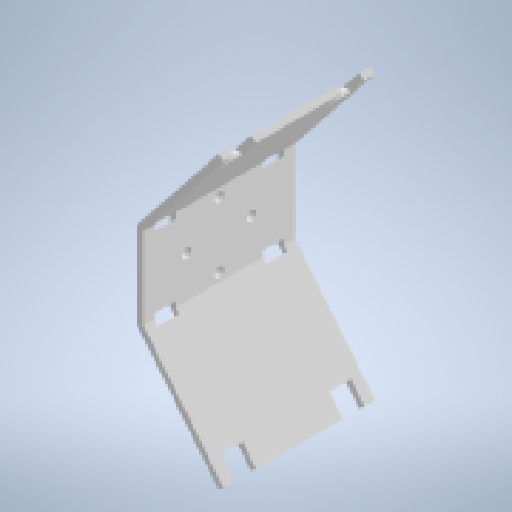
# Autodesk Inventor part: onTubeFixation
Saved by Autodesk Inventor 2024 (Build 280153000, 153)
## iProperties
Created: 2023-07-05
Part Number: onTubeFixation
Material: Generic
Document SubType Name: Sheet Metal
Designer: pablo
Density: 1 g/cm^3
Sheet Metal Rule: Default_mm
Appearance: Default
Author: pablo
Autodesk Inventor part; units mm, degrees
sketch "Sketch2" plane through (0, 0, 0) normal (0, 0, 1) x (1, 0, 0)
  line L0 (0, 0) -> (-40, 50)
  line L1 (-40, 50) -> (-40, 90)
  line L2 (-40, 90) -> (0, 140)
  line L3 (0, 140) -> (0, 0)
  line L4 (-2.3426, 137.0717) -> (0, 135.1977)
  line L5 (-2.3426, 2.9283) -> (0, 4.8023)
  dimension "d4" = 40
  dimension "d5" = 50
  dimension "d6" = 50
  dimension "d7" = 40
  dimension "d11" = 3
  dimension "d12" = 3
  constraints: 12 end point, 4 point on line, 2 perpendicular, 1 parallel, 1 vertical
  measures "d4" distance between parallel lines of L3 L1
  measures "d5" vertical distance of L2.end L1.end
  measures "d6" vertical distance of L0.start L0.end
  measures "d7" distance of L1.end L0.end
  measures "d11" distance of L4.start L4.end
  measures "d12" distance of L5.start L5.end
extrude "Extrusion2" add sketch "Sketch2" along normal mid plane 70 contours L0 L1 L2 L4 L3 L5
shell "Shell1" thickness 3 removed faces 5 at (-13.3333, 63.3333, -35) at (0, 91.7326, 11.6667) at (-13.3333, 63.3333, 35) at (-0.7809, 135.8224, -11.6667) at (-0.7809, 4.1776, 11.6667)
sketch "Sketch4" plane through (-2.3426, 2.9283, -35) normal (-0.7808688, -0.624695, 0) x (0, 0, 1)
  line L0 (0, 0) -> (70, 0) projected
  line L1 (5, 0) -> (15, 0)
  line L2 (15, 0) -> (15, 10)
  line L3 (15, 10) -> (5, 10)
  line L4 (5, 10) -> (5, 0)
  line L5 (55, 0) -> (65, 0)
  line L6 (65, 0) -> (65, 10)
  line L7 (65, 10) -> (55, 10)
  line L8 (55, 10) -> (55, 0)
  line L9 (70, 60.2812) -> (70, 0) projected
  line L10 (0, 0) -> (0, 60.2812) projected
  point P0 (35, -3.75)
  point P1 (70, 54.2734)
  point P2 (0, 54.2734)
  dimension "d54" = 10
  dimension "d55" = 10
  dimension "d56" = 5
  dimension "d57" = 5
  dimension "d58" = 10
  dimension "d59" = 10
  constraints: 16 end point, 4 parallel, 2 horizontal, 2 perpendicular, 2 point on line
  measures "d54" distance between parallel lines of L4 L2
  measures "d55" distance between parallel lines of L6 L8
  measures "d56" distance between parallel lines of L9 L6
  measures "d57" distance between parallel lines of L10 L4
  measures "d58" distance between parallel lines of L0 L3
  measures "d59" distance between parallel lines of L0 L7
extrude "Extrusion3" cut sketch "Sketch4" against normal through all
sketch "Sketch5" plane through (-2.3426, 137.0717, -35) normal (-0.7808688, 0.624695, 0) x (0, 0, 1)
  line L0 (0, 0) -> (70, 0) projected
  line L1 (65, 0) -> (55, 0)
  line L2 (55, 0) -> (55, -10)
  line L3 (55, -10) -> (65, -10)
  line L4 (65, -10) -> (65, 0)
  line L5 (5, 0) -> (15, 0)
  line L6 (15, 0) -> (15, -10)
  line L7 (15, -10) -> (5, -10)
  line L8 (5, -10) -> (5, 0)
  line L9 (0, -60.2812) -> (0, 0) projected
  line L10 (70, 0) -> (70, -60.2812) projected
  point P0 (35, -105.5716)
  point P1 (0, -54.2734)
  point P2 (70, -54.2734)
  point P3 (15, 0)
  point P4 (55, 0)
  dimension "d62" = 5
  dimension "d63" = 5
  dimension "d64" = 10
  dimension "d65" = 10
  dimension "d66" = 10
  constraints: 16 end point, 4 parallel, 3 point on line, 2 horizontal, 2 perpendicular
  measures "d62" distance between parallel lines of L9 L8
  measures "d63" distance between parallel lines of L10 L4
  measures "d64" distance between parallel lines of L2 L4
  measures "d65" distance between parallel lines of L8 L6
  measures "d66" distance between parallel lines of L0 L3
extrude "Extrusion4" cut sketch "Sketch5" against normal through all
fillet "Fillet3" radius 3 4 edges at (-8.5896, 129.2631, -25) (-8.5896, 129.2631, 25) (-8.5896, 10.7369, -25) (-8.5896, 10.7369, 25)
ref_plane "Work Plane1" through (-40, 90, -35) normal (0.3310069, 0.9436283, 0) x (0, 0, -1)
ref_plane "Work Plane2" through (-40, 50, -35) normal (0.3310069, -0.9436283, 0) x (0, 0, 1)
sketch "Sketch8" plane through (-40, 90, -35) normal (0.3310069, 0.9436283, 0) x (0, 0, -1)
  line L0 (0, 0) -> (-70, 0) projected
  line L1 (-65, 0) -> (-55, 0)
  line L2 (-55, 0) -> (-55, -4)
  line L3 (-55, -4) -> (-65, -4)
  line L4 (-65, -4) -> (-65, 0)
  line L5 (-70, -15.7228) -> (-70, -3.1792) projected
  line L6 (-15, 0) -> (-5, 0)
  line L7 (-5, 0) -> (-5, -4)
  line L8 (-5, -4) -> (-15, -4)
  line L9 (-15, -4) -> (-15, 0)
  line L10 (0, -13.2403) -> (0, 0) projected
  point P0 (-35, -67.5358)
  dimension "d87" = 10
  dimension "d88" = 5
  dimension "d89" = 4
  dimension "d90" = 5
  dimension "d91" = 10
  dimension "d92" = 4
  constraints: 16 end point, 4 parallel, 2 horizontal, 2 perpendicular, 2 point on line
  measures "d87" distance between parallel lines of L2 L4
  measures "d88" distance between parallel lines of L5 L4
  measures "d89" distance between parallel lines of L3 L0
  measures "d90" distance between parallel lines of L10 L7
  measures "d91" distance between parallel lines of L7 L9
  measures "d92" distance between parallel lines of L0 L8
extrude "Extrusion5" cut sketch "Sketch8" along normal through all both and the other way through all
ref_plane "Work Plane3" through (-56, 70, -20) normal (0, 1, 0) x (0, 0, -1)
mirror "Mirror1" about plane through (-56, 70, -20) normal (0, 1, 0) of "Extrusion5"
sketch "Sketch9" plane through (-40, 50, 35) normal (-1, 0, 0) x (0, 0, 1)
  line L0 (-70, 0) -> (-70, 40) projected
  line L1 (0, 40) -> (0, 0) projected
  line L2 (-70, 0) -> (0, 40)
  line L3 (-70, 40) -> (-65, 40) projected
  line L4 (0, 0) -> (-70, 40)
  line L5 (-35, 20) -> (0, 20)
  line L6 (-35, 20) -> (-70, 20)
  line L7 (-35, 20) -> (-35, 40)
  line L8 (-55, 40) -> (-15, 40) projected
  line L9 (-35, 20) -> (-35, 0)
  line L10 (-15, 0) -> (-55, 0) projected
  line L11 (-50, 20) -> (-35, 35)
  line L12 (-20, 20) -> (-35, 5)
  line L13 (-35, 5) -> (-50, 20)
  line L14 (-20, 20) -> (-35, 35)
  point P0 (-35, -50)
  dimension "d95" = 30
  dimension "d96" = 30
  constraints: 20 end point, 5 midpoint, 4 point on line, 3 perpendicular
  measures "d95" distance of L11.end L12.end
  measures "d96" distance of L12.start L11.start
hole "Hole2" at (-40, 70, -15) at (-40, 85, 0) at (-40, 70, 15) at (-40, 55, 0) direction (1, 0, 0) diameter 4.2 depth 5
equation "\"d102\" = Thickness"
equation "\"BendRadius\" = Thickness"
equation "\"BendReliefWidth\" = Thickness"
equation "\"BendReliefDepth\" = 0.5 * Thickness"
equation "\"TransitionRadius\" = BendRadius"
equation "\"JacobiRadiusSize\" = BendRadius"
equation "\"GapSize\" = Thickness"
equation "\"d13\" = Thickness"
equation "\"Thickness\" = 5"
body "Solid2"
